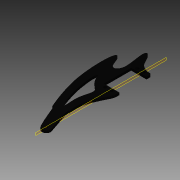
# Autodesk Inventor part: tibia
Saved by Autodesk Inventor 2015 (Build 190159000, 159)
## iProperties
Created: 2015-01-27
Part Number: tibia
Material: ABS Plastic
Document SubType Name: Modeling
Designer: Rafi Kurnia Putra
Density: 1.06 g/cm^3
Appearance: Smooth - Black
Mass: 14.699 g
Surface Area: 104.017 cm^2
Volume: 13.867 cm^3
Author: Rafi Kurnia Putra
Autodesk Inventor part; units mm, degrees
ref_plane "YZ Plane" through (0, 0, 0) normal (1, 0, 0) x (0, 1, 0)
ref_plane "XZ Plane" through (0, 0, 0) normal (0, 1, 0) x (-1, 0, 0)
ref_plane "XY Plane" through (0, 0, 0) normal (0, 0, 1) x (1, 0, 0)
sketch "Sketch1" plane through (0, 0, 0) normal (0, 0, 1) x (1, 0, 0)
  spline S0 degree 3 poles (28.5231, 4.0546) (28.5122, 3.8777) (28.4911, 3.536) (28.4296, 3.0423) (28.3496, 2.5831) (28.2534, 2.1542) (28.1433, 1.7518) (28.0229, 1.3715) (27.8944, 1.0097) (27.7616, 0.6618) (27.6279, 0.3271) (27.5396, 0.1075) (27.4969, 0) knots 0 0 0 0 0.126355 0.244108 0.354546 0.458642 0.557466 0.651949 0.743008 0.831228 0.917493 1 1 1 1
  line L0 (28.5364, 4.6271) -> (28.5231, 4.0546)
  spline S1 degree 3 poles (-23.3496, 0) (-23.5596, 1.2846) (-24.0562, 4.5179) (-24.7325, 9.6962) (-25.3412, 15.4949) (-25.8019, 21.1836) (-26.1178, 26.6913) (-26.2938, 31.9464) (-26.334, 36.8778) (-26.2429, 41.414) (-26.0271, 45.4846) (-25.6884, 49.0186) (-25.2468, 51.9498) (-24.6777, 54.2125) (-24.0754, 55.7888) (-23.2476, 56.6327) (-22.505, 56.6995) (-21.9625, 56.5517) (-21.4825, 56.2045) (-21.0506, 55.7047) (-20.6464, 55.0659) (-20.2596, 54.3032) (-19.8805, 53.432) (-19.5021, 52.4684) (-19.1154, 51.4296) (-18.7137, 50.3325) (-18.2883, 49.1949) (-17.832, 48.034) (-17.3361, 46.8673) (-16.7931, 45.7122) (-16.1948, 44.586) (-15.6089, 43.6313) (-15.0532, 42.8382) (-14.5538, 42.185) (-14.0248, 41.5499) (-13.4716, 40.9391) (-12.8992, 40.3596) (-12.3127, 39.8177) (-11.7174, 39.3202) (-11.1182, 38.8737) (-10.5205, 38.4843) (-9.9288, 38.1591) (-9.3484, 37.9042) (-8.7834, 37.7267) (-8.238, 37.6326) (-7.7172, 37.6324) (-7.2224, 37.7286) (-6.4152, 38.1342) (-5.3985, 38.9168) (-4.2272, 40.0742) (-3.2961, 41.391) (-2.5764, 42.8393) (-2.0505, 44.4149) (-1.6978, 46.1099) (-1.4984, 47.9194) (-1.4336, 49.8385) (-1.4848, 51.8623) (-1.6347, 53.9859) (-1.8653, 56.2043) (-2.1596, 58.5118) (-2.4992, 60.9034) (-2.8674, 63.3732) (-3.2464, 65.9158) (-3.5664, 68.1668) (-3.8215, 70.0724) (-4.013, 71.5797) (-4.1779, 72.9988) (-4.3125, 74.3273) (-4.412, 75.5631) (-4.4736, 76.7037) (-4.4924, 77.7473) (-4.4652, 78.6917) (-4.3869, 79.535) (-4.2545, 80.2758) (-4.0623, 80.913) (-3.805, 81.4458) (-3.4729, 81.8701) (-3.0598, 82.1796) (-2.5651, 82.3579) (-2.0087, 82.4253) (-1.3965, 82.3012) (-0.8113, 81.9154) (-0.2469, 81.3444) (0.3151, 80.5978) (0.8842, 79.6972) (1.4674, 78.6612) (2.0715, 77.5121) (2.702, 76.2711) (3.3657, 74.9608) (4.0685, 73.6031) (4.8168, 72.2207) (5.6168, 70.8358) (6.4749, 69.4707) (7.3984, 68.1483) (8.3914, 66.8886) (9.4635, 65.7294) (10.5733, 64.6742) (11.6739, 63.7035) (12.7645, 62.8288) (13.8421, 62.0439) (14.9058, 61.3452) (15.9546, 60.7287) (16.987, 60.1902) (18.0021, 59.7258) (18.9984, 59.3311) (19.9751, 59.0025) (20.9306, 58.7354) (21.8641, 58.5267) (22.7741, 58.3706) (23.6596, 58.2656) (24.5193, 58.2023) (25.2049, 58.1938) (25.7184, 58.186) (26.0625, 58.156) (26.3869, 58.1066) (26.6913, 58.0364) (26.975, 57.9448) (27.2375, 57.8314) (27.478, 57.6958) (27.6958, 57.5371) (27.8904, 57.3553) (28.0607, 57.1497) (28.2063, 56.9203) (28.3261, 56.6666) (28.4204, 56.3888) (28.4873, 56.086) (28.5292, 55.7584) (28.534, 55.5314) (28.5364, 55.414) knots 0.254722 0.254722 0.254722 0.254722 0.271315 0.296419 0.321287 0.345633 0.369168 0.391606 0.412655 0.432027 0.449436 0.464605 0.477268 0.487197 0.494265 0.498771 0.50116 0.503403 0.505815 0.508584 0.511786 0.515425 0.519476 0.523892 0.528622 0.533605 0.538785 0.544103 0.549506 0.554941 0.560369 0.565753 0.569207 0.572709 0.57623 0.57974 0.58321 0.58661 0.589913 0.593093 0.596129 0.598998 0.601689 0.604196 0.606528 0.608713 0.610804 0.612882 0.620155 0.627058 0.633809 0.640606 0.647605 0.654923 0.662636 0.670784 0.679383 0.688432 0.697915 0.70781 0.718085 0.728707 0.739642 0.750856 0.75769 0.764151 0.770225 0.775902 0.781172 0.786027 0.790462 0.794474 0.798065 0.801249 0.804052 0.806524 0.808749 0.810856 0.81301 0.815378 0.817925 0.820785 0.824166 0.82813 0.83267 0.83774 0.843279 0.849217 0.855484 0.862003 0.868704 0.875519 0.882387 0.889251 0.89607 0.902815 0.909357 0.915583 0.921514 0.927169 0.932568 0.937728 0.942668 0.947402 0.951949 0.95632 0.960529 0.964588 0.968506 0.97229 0.975949 0.979485 0.981027 0.982492 0.983884 0.985206 0.986469 0.987677 0.988844 0.989981 0.991104 0.992229 0.993375 0.994558 0.995797 0.997108 0.998504 1 1 1 1
  spline S2 degree 3 poles (-11.7382, 0) (-11.7408, 0.0214) (-11.8537, 0.9472) (-12.0561, 2.7409) (-12.2937, 5.3299) (-12.4518, 7.7565) (-12.519, 9.9679) (-12.4833, 11.9122) (-12.337, 13.5384) (-12.0678, 14.8092) (-11.7107, 15.5993) (-11.3088, 15.9793) (-10.9531, 15.963) (-10.6703, 15.6984) (-10.3895, 15.2959) (-10.0852, 14.7302) (-9.75, 14.022) (-9.3744, 13.1832) (-8.9516, 12.2312) (-8.4717, 11.1834) (-7.9277, 10.0566) (-7.3101, 8.8684) (-6.611, 7.636) (-5.8206, 6.3773) (-4.9311, 5.1094) (-3.9341, 3.8489) (-2.9017, 2.7136) (-1.909, 1.7266) (-1.0284, 0.8963) (-0.396, 0.3372) (-0.0594, 0.0503) (0, 0) knots 0 0 0 0 0.001794 0.077439 0.14988 0.21766 0.279336 0.333546 0.379025 0.414811 0.440809 0.450487 0.458087 0.467745 0.48131 0.499074 0.520875 0.54642 0.575368 0.607373 0.642106 0.679254 0.718539 0.759722 0.802612 0.847081 0.893064 0.929924 0.963288 0.993536 1 1 1 1
  line L1 (25.7361, 9.2947) -> (5.1113, 9.2943)
  line L2 (5.1113, 9.2943) -> (5.111, 50.7365)
  line L3 (5.111, 50.7365) -> (25.7356, 50.7361)
  spline S3 degree 3 poles (-23.3496, 0) (-22.2299, -6.8529) (-20.6397, -14.7032) (-13.6938, -37.2211) (-10.14, -46.5601) (-7.4055, -53.2168) knots 0.000001 0.000001 0.000001 0.000001 2.083126 2.083126 3.800874 3.800874 3.800874 3.800874
  spline S4 degree 3 poles (14.944, -53.2168) (14.7208, -51.9235) (14.3261, -49.6117) (13.9047, -44.2854) (13.7783, -41.8254) (14.0159, -36.757) (14.4834, -32.3937) (17.9139, -21.3639) (19.7308, -16.8534) (22.0939, -11.617) (22.658, -10.4089) (23.2956, -9.0607) (23.7019, -8.206) (24.492, -6.6157) (24.7448, -6.1165) (25.2637, -5.0274) (25.4661, -4.5883) (26.2249, -3.1125) (26.5541, -2.7392) (26.9677, -1.7598) (26.9376, -1.6424) (27.2417, -0.6479) (27.4007, -0.2421) (27.4969, 0) knots 0.000001 0.000001 0.000001 0.000001 0.393736 0.393736 0.639098 0.639098 0.904888 0.904888 1.083033 1.083033 1.13024 1.13024 1.155458 1.155458 1.173487 1.173487 1.185531 1.185531 1.214726 1.214726 1.234664 1.234664 1.249345 1.249345 1.249345 1.249345
  spline S5 degree 3 poles (-11.7382, 0) (-11.1037, -5.2) (-10.1194, -11.112) (-8.3888, -19.3849) (-7.0539, -24.4927) (-3.3184, -36.6072) (-1.4427, -42.1645) (1.0735, -47.6165) (1.5831, -48.3867) (2.0889, -49.0978) (2.3165, -49.3581) (2.5304, -49.5783) (2.63, -49.6662) (2.8368, -49.7882) (2.9352, -49.8262) (3.1285, -49.8602) (3.2196, -49.8628) (3.3667, -49.8387) (3.4267, -49.8201) (3.5239, -49.7669) (3.5674, -49.7338) (3.6552, -49.6275) (3.6903, -49.5639) (3.7589, -49.4087) (3.8049, -49.2813) (3.8704, -48.9087) (3.9147, -48.5693) (3.9591, -46.7677) (3.8331, -44.9985) (3.3073, -37.4403) (2.9716, -31.7043) (4.5041, -22.4163) (6.163, -17.2219) (7.0491, -12.6663) (7.1665, -11.9578) (7.3493, -10.309) (7.4238, -8.9827) (7.1059, -7.5419) (6.9022, -6.6748) (4.6386, -3.1087) (2.9829, -2.5273) (0, 0) knots 0.000001 0.000001 0.000001 0.000001 1.571558 1.571558 2.718882 2.718882 3.544275 3.544275 3.937447 3.937447 4.344722 4.344722 4.647881 4.647881 4.899345 4.899345 5.101719 5.101719 5.244575 5.244575 5.358606 5.358606 5.476932 5.476932 5.645003 5.645003 5.780754 5.780754 6.07526 6.07526 6.779551 6.779551 7.366129 7.366129 7.470241 7.470241 7.612697 7.612697 7.639863 7.639863 7.692175 7.692175 7.692175 7.692175
  spline S6 degree 3 poles (-5.7428, -57.1863) (-6.1455, -56.2349) (-6.7048, -54.9138) (-7.2529, -53.5881) (-7.4055, -53.2168) knots 0 0 0 0 0.720187 1 1 1 1
  line L4 (-5.7428, -57.1863) -> (-4.5199, -60.0164)
  line L5 (-4.5199, -60.0164) -> (-3.0104, -59.484)
  spline S7 degree 3 poles (12.0779, -93.6212) (11.7449, -92.9916) (11.0623, -91.7012) (10.0686, -89.6953) (9.0632, -87.5918) (8.0534, -85.4012) (7.0384, -83.1383) (6.0212, -80.8161) (5.0022, -78.4487) (3.9844, -76.0491) (2.968, -73.6315) (1.9557, -71.2092) (0.9481, -68.796) (-0.0522, -66.4054) (-1.0448, -64.0512) (-2.0258, -61.7464) (-2.685, -60.2317) (-3.0104, -59.484) knots 0 0 0 0 0.057236 0.117297 0.179852 0.244573 0.311117 0.379138 0.44829 0.518223 0.588584 0.659024 0.729185 0.798716 0.867263 0.934475 1 1 1 1
  line L6 (12.0779, -93.6212) -> (12.9977, -95.2825)
  ellipse E0 centre (18.5814, -92.1925) end of major axis (24.9635, -92.1925) minor radius 6.3804 (12.9977, -95.2825) -> (24.6279, -90.1509) ccw
  line L7 (24.6279, -90.1509) -> (22.1409, -82.7892)
  spline S8 degree 3 poles (13.4806, -53.8275) (13.7067, -55.0284) (14.0921, -56.9051) (14.6845, -59.386) (15.3236, -61.8401) (16.1992, -64.8707) (17.3372, -68.4662) (18.5286, -72.0405) (20.1367, -76.8076) (21.3388, -80.3969) (22.1409, -82.7892) knots 0 0 0 0 0.119755 0.179633 0.23951 0.359266 0.479021 0.598776 0.718531 0.958042 0.958042 0.958042 0.958042
  line L8 (13.4806, -53.8275) -> (14.9577, -53.2966)
  line L9 (14.9577, -53.2966) -> (14.944, -53.2168)
  circle A0 centre (18.5814, -92.1925) radius 1.75
  line L10 (25.7356, 50.7361) -> (28.5364, 50.7361)
  line L11 (25.7361, 9.2947) -> (28.5364, 9.2947)
  line L12 (28.5364, 55.414) -> (28.5364, 50.7361)
  line L13 (28.5364, 9.2947) -> (28.5364, 4.6271)
  circle A1 centre (10.5215, 54.6091) radius 2.2352
  circle A2 centre (20.3255, 54.5253) radius 2.2352
  circle A3 centre (10.5215, 5.4093) radius 2.2352
  circle A4 centre (20.3259, 5.4093) radius 2.2352
  point P0 (0, 0)
  point P1 (5.1111, 9.2945)
  dimension "d0" = 3.5
  dimension "d9" = 9.8044
  dimension "d10" = 4.4704
  dimension "d11" = 4.4704
  dimension "d12" = 4.4704
  dimension "d13" = 9.8044
  dimension "d14" = 49.1998
  dimension "d15" = 49.116
  constraints: 28 end point, 5 centre point, 2 coincident, 2 perpendicular, 1 horizontal, 1 vertical alignment, 25 other
  measures "d0" diameter of A0
  measures "d9" distance of A2.centre A1.centre
  measures "d10" diameter of A1
  measures "d11" diameter of A3
  measures "d12" diameter of A4
  measures "d13" distance of A4.centre A3.centre
  measures "d14" distance of A3.centre A1.centre
  measures "d15" distance of A4.centre A2.centre
extrude "Extrusion2" add sketch "Sketch1" along normal mid plane 3.5
body "Solid2"
